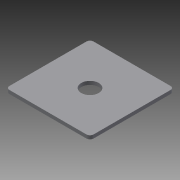
# Autodesk Inventor part: motorMount
Saved by Autodesk Inventor 2013 (Build 170138000, 138)
## iProperties
Created: 2012-12-12
Part Number: motorMount
Material: Generic
Document SubType Name: Modeling
Designer: istvan.burbank
Density: 1 g/cm^3
Author: istvan.burbank
Autodesk Inventor part; units mm, degrees
ref_plane "YZ Plane" through (0, 0, 0) normal (1, 0, 0) x (0, 1, 0)
ref_plane "XZ Plane" through (0, 0, 0) normal (0, 1, 0) x (-1, 0, 0)
ref_plane "XY Plane" through (0, 0, 0) normal (0, 0, 1) x (1, 0, 0)
sketch "Sketch1" plane through (0, 0, 0) normal (0, 1, 0) x (-1, 0, 0)
  line L0 (3.175, 0) -> (73.025, 0)
  line L1 (76.2, 3.175) -> (76.2, 73.025)
  line L2 (73.025, 76.2) -> (3.175, 76.2)
  line L3 (0, 73.025) -> (0, 3.175)
  arc A0 (3.175, 76.2) -> (0, 73.025) centre (3.175, 73.025) ccw
  arc A1 (76.2, 73.025) -> (73.025, 76.2) centre (73.025, 73.025) ccw
  arc A2 (73.025, 0) -> (76.2, 3.175) centre (73.025, 3.175) ccw
  arc A3 (0, 3.175) -> (3.175, 0) centre (3.175, 3.175) ccw
  point P0 (0, 0)
  point P1 (76.2, 76.2)
  point P2 (76.2, 0)
  point P3 (0, 76.2)
  dimension "d0" = 76.2
  dimension "d1" = 76.2
  dimension "d13" = 3.175
  constraints: 8 end point, 8 point on circle, 8 point on line, 8 tangent, 4 centre point, 3 equal radius, 2 parallel, 1 horizontal, 1 perpendicular
  measures "d0" distance of point (0, 76.2) point (76.2, 76.2)
  measures "d1" distance of point (76.2, 76.2) point (76.2, 0)
  measures "d13" radius of A0
extrude "Extrusion1" add sketch "Sketch1" along normal blind 3.175
sketch "Sketch2" plane through (0, 3.175, 0) normal (0, 1, 0) x (1, 0, 0)
  line L0 (-3.175, 0) -> (-73.025, 0) projected
  line L1 (-76.2, -3.175) -> (-76.2, -73.025) projected
  point P0 (0, 0)
  point P1 (-76.2, 0)
  point P2 (-76.2, -76.2)
  point P3 (-38.1, -38.1)
  dimension "d4" = 38.1
  dimension "d5" = 38.1
  measures "d4" distance from line of point (-38.1, -38.1) L1
  measures "d5" distance from line of L0 point (-38.1, -38.1)
hole "Hole1" at (-38.1, 3.175, 38.1) direction (0, -1, 0) diameter 15.875 end through all
body "Solid1"
